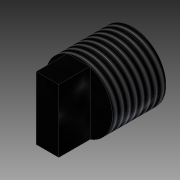
# Autodesk Inventor part: voet
Saved by Autodesk Inventor 2015 (Build 190159000, 159)
## iProperties
Created: 2016-01-04
Part Number: voet
Material: Generic
Document SubType Name: Modeling
Designer: david
Density: 1 g/cm^3
Appearance: Black
Mass: 2.6191 g
Surface Area: 11.8728 cm^2
Volume: 2.6191 cm^3
Author: david
Autodesk Inventor part; units mm, degrees
ref_plane "YZ Plane" through (0, 0, 0) normal (1, 0, 0) x (0, 1, 0)
ref_plane "XZ Plane" through (0, 0, 0) normal (0, 1, 0) x (-1, 0, 0)
ref_plane "XY Plane" through (0, 0, 0) normal (0, 0, 1) x (1, 0, 0)
sketch "Sketch1" plane through (0, 0, 0) normal (0, 1, 0) x (-1, 0, 0)
  circle A0 centre (0, 0) radius 7.5
  dimension "d0" = 15
  constraints: 1 centre point, 1 coincident
  measures "d0" diameter of A0
extrude "Extrusion1" add sketch "Sketch1" along normal blind 12
sketch "Sketch2" plane through (0, 0, 0) normal (0, -1, 0) x (1, 0, 0)
  circle A0 centre (0, 0) radius 7.5 projected
  line L0 (-2.5206, -7.0638) -> (2.5206, -7.0638)
  line L1 (2.5206, -7.0638) -> (2.5206, 7.0638)
  line L2 (2.5206, 7.0638) -> (-2.5206, 7.0638)
  line L3 (-2.5206, 7.0638) -> (-2.5206, -7.0638)
  line L4 (-2.5206, -7.0638) -> (2.5206, 7.0638) construction
  line L5 (2.5206, -7.0638) -> (-2.5206, 7.0638) construction
  constraints: 12 end point, 2 midpoint, 2 parallel, 1 horizontal, 1 perpendicular, 2 other
extrude "Extrusion2" add sketch "Sketch2" along normal blind 7 contours L1 L0 L3 L2
thread "Thread1" size "M15x1.5" class "6g" standard "ANSI Metric M Profile" full length
body "Solid1"
